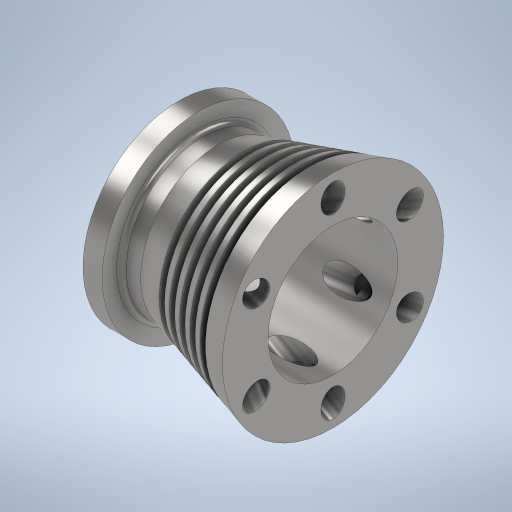
# Autodesk Inventor part: gehäuse_winkel_bohrung
Saved by Autodesk Inventor 2024 (Build 280153000, 153)
## iProperties
Created: 2024-03-08
Part Number: gehäuse_winkel_bohrung
Material: Stahl, weich
Document SubType Name: Modeling
Designer: ffogue
Density: 7.85 g/cm^3
Appearance: Halbpoliert
Author: ffogue
Autodesk Inventor part; units mm, degrees
note: some values were not read from the file. Chosen so that the rebuilt part matches the saved one: direction of "Bohrung1".
sketch "Skizze1" plane through (0, 0, 0) normal (0, 0, 1) x (1, 0, 0)
  line L0 (0, 0) -> (32, 0)
  line L1 (0, 0) -> (0, 20)
  line L2 (0, 20) -> (4, 20)
  line L3 (4, 20) -> (4, 16)
  line L4 (4, 16) -> (8, 16)
  line L5 (8, 16) -> (32, 23)
  line L6 (32, 23) -> (32, 0)
  dimension "d0" = 32
  dimension "d1" = 46
  dimension "d2" = 4
  dimension "d3" = 40
  dimension "d4" = 32
  dimension "d5" = 4
  constraints: 14 end point, 3 perpendicular, 2 vertical, 1 coincident, 1 horizontal
  measures "d0" distance of L0.start L0.end
  measures "d1" diameter of L5.end L0
  measures "d2" distance between parallel lines of L3 L1
  measures "d3" diameter of L2 L0
  measures "d4" diameter of L3.end L0
  measures "d5" distance from line of L4.end L3
revolve "Umdrehung1" add sketch "Skizze1" angle 360 about axis through (0, 0, 0) along (1, 0, 0)
sketch "Skizze2" plane through (0, 0, 0) normal (-1, 0, 0) x (0, 0, 1)
  circle A0 centre (0, 0) radius 20 projected
  constraints: 1 coincident
hole "Bohrung1" at (0, 0, 0) direction (1, 0, 0) diameter 27 depth 32
ref_plane "Arbeitsebene2" through (0, 0, 0) normal (0, 0, 1) x (1, 0, 0)
sketch "Skizze4" plane through (0, 0, 0) normal (0, 0, 1) x (1, 0, 0)
  line L0 (8, 16) -> (32, 23) projected
  line L1 (27, 21.5417) -> (27, 16)
  line L2 (27, 16) -> (25.5, 16)
  line L3 (25.5, 16) -> (25.5, 21.1042)
  line L4 (32, -23) -> (32, 23) projected
  line L5 (0, 0) -> (36.6178, 0)
  point P0 (25.5, 18.5521)
  dimension "d16" = 5
  dimension "d17" = 1.5
  dimension "d19" = 32
  constraints: 8 end point, 2 perpendicular, 2 point on line, 1 horizontal, 1 midpoint, 1 vertical
  measures "d16" distance between parallel lines of L4 L1
  measures "d17" distance from line of L1 point (25.5, 18.552)
  measures "d19" diameter of L2 L5
revolve "Umdrehung2" cut sketch "Skizze4" angle 360 about axis through (0, 0, 0) along (1, 0, 0)
pattern_linear "Rechteckige Anordnung1" count 5 spacing 3 along (-1, 0, 0) of "Umdrehung2"
ref_plane "Arbeitsebene4" through (0, 0, 0) normal (0, 1, 0) x (-1, 0, 0)
sketch "Skizze6" plane through (0, 0, 0) normal (0, 1, 0) x (-1, 0, 0)
  line L0 (0, 0) -> (-34.641, -20) construction
  line L1 (0, 13.5) -> (0, -13.5) projected
  dimension "d26" = 60
  dimension "d27" = 40
  constraints: 2 end point
  measures "d26" angle of L1 L0
  measures "d27" distance of L0.start L0.end
ref_plane "Arbeitsebene5" through (34.641, 0, -20) normal (0, 0, -1) x (-1, 0, 0)
hole "Bohrung2" at (34.641, 0, -20) direction (-0.8660254, 0, 0.5) diameter 5 end through all
pattern_circular "Runde Anordnung1" count 6 over 360 about axis through (72.4983, 0, 0) along (-1, 0, 0) of "Bohrung2"
fillet "Rundung1" radius 1 1 edges at (4, -16, 0)
